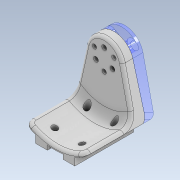
# Autodesk Inventor part: shank_thigh_connector_v3
Saved by Autodesk Inventor 2020 (Build 240168000, 168)
## iProperties
Created: 2021-01-06
Part Number: shank_thigh_connector_v3
Material: PC/ABS Plastic
Document SubType Name: Modeling
Designer: DELL
Density: 0.357273 g/cm^3
Appearance: Clear - Blue
Author: DELL
Autodesk Inventor part; units mm, degrees
ref_plane "YZ Plane" through (0, 0, 0) normal (1, 0, 0) x (0, 1, 0)
ref_plane "XZ Plane" through (0, 0, 0) normal (0, 1, 0) x (-1, 0, 0)
sketch "Sketch1" plane through (0, 0, 0) normal (0, 0, 1) x (1, 0, 0)
  circle A0 centre (0, 0) radius 19
  line L0 (-18.5454, 4.1315) -> (-30, -47.2864)
  line L1 (18.5454, 4.1315) -> (30, -47.2864)
  line L2 (9.9593, -5.75) -> (0, 0) construction
  circle A1 centre (8.4134, -4.8575) radius 2.5
  line L3 (0, 0) -> (9.9593, 5.75) construction
  line L4 (0, 0) -> (-9.9593, -5.75) construction
  circle A2 centre (-8.4134, -4.8575) radius 2.5
  circle A3 centre (0, 0) radius 9.715 construction
  circle A4 centre (0, 0) radius 11.5 construction
  circle A5 centre (0, 9.715) radius 2.5
  line L5 (0, 0) -> (-9.9593, 5.75) construction
  line L6 (11.5, 0) -> (-11.5, 0) construction
  circle A6 centre (-9.9593, 5.75) radius 4
  circle A7 centre (-9.9593, 5.75) radius 2.25
  line L7 (0, -48.5721) -> (0, 22.5) construction
  circle A8 centre (0, -11.5) radius 2.25
  circle A9 centre (0, -11.5) radius 4
  circle A10 centre (9.9593, 5.75) radius 4
  circle A11 centre (9.9593, 5.75) radius 2.25
  arc A12 (-29.0707, -43.1149) -> (29.0707, -43.1149) centre (0, 0) ccw
  arc A13 (-30, -47.2864) -> (30, -47.2864) centre (0, 0) ccw
  line L8 (30, -47.2864) -> (30, -60)
  line L9 (30, -60) -> (-30, -60)
  line L10 (-30, -60) -> (-30, -47.2864)
  line L11 (8, -55.4256) -> (8, -60)
  line L12 (-8, -55.4256) -> (-8, -60)
  line L13 (20, -52.3068) -> (20, -60)
  line L14 (-20, -52.3068) -> (-20, -60)
  point P0 (0, 11.4686)
  point P1 (0, 11.4686)
  point P2 (11.5, 0)
  point P3 (-11.5, 0)
  point P4 (0, -56)
  point P5 (0, -56)
  dimension "d18" = 23
  dimension "d0" = 38
  dimension "d17" = 19.43
  dimension "d19" = 30
  dimension "d20" = 30
  dimension "d21" = 4.5
  dimension "d22" = 8
  dimension "d23" = 5
  dimension "d24" = 104
  dimension "d25" = 112
  dimension "d48" = 60
  dimension "d84" = 16
  dimension "d85" = 4.5744
  dimension "d86" = 22
  dimension "d104" = 60
  dimension "d116" = 40
  constraints: 28 end point, 14 point on circle, 13 centre point, 12 point on line, 10 coincident, 6 equal radius, 6 perpendicular, 2 tangent, 2 vertical, 19 other
  measures "d0" diameter of A0
  measures "d17" diameter of A3
  measures "d19" angle to the sketch x axis of L5
  measures "d20" angle to the sketch x axis of L4
  measures "d21" diameter of A11
  measures "d22" diameter of A10
  measures "d23" diameter of A5
  measures "d24" diameter of A12
  measures "d25" diameter of A13
  measures "d48" distance of L1.end L0.end
  measures "d84" distance between parallel lines of L11 L12
  measures "d85" distance of L11.start L11.end
  measures "d86" distance between parallel lines of L8 L11
  measures "d104" distance from line of A0.centre L9
  measures "d116" distance between parallel lines of L14 L13
extrude "Extrusion1" add sketch "Sketch1" against normal blind 10 contours A0 | A0 L1 A12 L0 | L1 A13 L0 A12 | A1 | A2 | A5 | A6 | A7 | A8 | A9 | A10 | A11
sketch "Sketch4" plane through (0, 0, 0) normal (1, 0, 0) x (0, 1, 0)
  line L0 (4.1315, -10) -> (19, -10) projected
  line L1 (-53, -13) -> (19, -10)
  line L2 (-53, -13) -> (-56, -10)
  line L3 (-53, -13) -> (0, -66)
  line L4 (0, -66) -> (-65, -66)
  line L5 (-65, -66) -> (-65, -1)
  line L6 (4.1315, 0) -> (4.1315, 0) projected
  line L7 (4.1315, 0) -> (4.1315, -10) projected
  line L8 (4.1315, -10) -> (4.1315, -10) projected
  line L9 (4.1315, 0) -> (4.1315, -10) projected
  line L10 (4.1315, 0) -> (-47.2864, 0) projected
  line L11 (-56, -10) -> (-47.2864, -10) projected
  line L12 (-56, -10) -> (19, -10)
  line L13 (-56, 0) -> (-56, -10) projected
  line L14 (-56, -10) -> (-65, -1)
  line L15 (-47.2864, 0) -> (-47.2864, 0) projected
  line L16 (-47.2864, 0) -> (-47.2864, -10) projected
  line L17 (-47.2864, -10) -> (-47.2864, -10) projected
  line L18 (-47.2864, 0) -> (-47.2864, -10) projected
  line L19 (-56, -10) -> (0, -10)
  line L20 (0, -10) -> (0, -66)
  line L21 (19, 0) -> (19, -10) projected
  dimension "d81" = 3
  dimension "d82" = 3
  dimension "d92" = 56
  dimension "d96" = 65
  constraints: 19 end point, 3 collinear, 3 point on line, 2 perpendicular, 1 horizontal
  measures "d81" horizontal distance of L1.start L2.end
  measures "d82" horizontal distance of L1.start L2.end
  measures "d92" distance of L13.end L19.end
  measures "d96" distance between parallel lines of L20 L5
extrude "Extrusion9" add sketch "Sketch4" along normal mid plane 60 contours L0 L1 L20 L12 | L20 L1 L2 L11 L12
extrude "Extrusion10" cut sketch "Sketch1" against normal blind 60 from surface at 0 contours A0 | A0 L1 A12 L0 | L1 A13 L0 A12 | A1 | A2 | A5 | A6 | A7 | A8 | A9 | A10 | A11 keep common part
revolve "Revolution1" cut sketch "Sketch4" angle 360 about axis through (0, 0, -10) along (0, 0, -1) contours L3 L4 L5 L14 L2
sketch "Sketch5" plane through (0, 0, 0) normal (0, 0, 1) x (1, 0, 0)
  arc A0 (-30, -47.2864) -> (30, -47.2864) centre (0, 0) ccw projected
  line L0 (8, -55.4256) -> (8, -60)
  line L1 (-8, -60) -> (-8, -55.4256)
  line L2 (0, 0) -> (0, -56) construction
  line L3 (-8, -60) -> (8, -60)
  line L4 (30, -47.2864) -> (30, -60)
  line L5 (30, -60) -> (8, -60)
  line L6 (-8, -60) -> (-30, -60)
  line L7 (-30, -60) -> (-30, -47.2864)
  line L8 (20, -52.3068) -> (20, -60)
  line L9 (-20, -52.3068) -> (-20, -60)
  line L10 (0, -56) -> (0, -60) construction
  dimension "d93" = 16
  dimension "d94" = 22
  dimension "d95" = 4.5744
  dimension "d105" = 60
  dimension "d117" = 40
  constraints: 22 end point, 5 point on circle, 3 perpendicular, 3 point on line, 3 vertical, 1 horizontal, 1 midpoint, 1 parallel, 2 other
  measures "d93" distance between parallel lines of L0 L1
  measures "d94" distance from line of L4.start L0
  measures "d95" distance of L0.start L0.end
  measures "d105" distance from line of point (0, 0) L3
  measures "d117" distance between parallel lines of L9 L8
extrude "Extrusion14" add sketch "Sketch5" against normal up to surface (10 mm away) contours A0 L1 L6 L9 | A0 L8 L5 L0
extrude "Extrusion11" cut sketch "Sketch1" against normal through all contours A7 | A8 | A11
extrude "Extrusion12" cut sketch "Sketch1" against normal blind 4 contours A1 | A2 | A5
ref_plane "Work Plane1" through (0, 0, -5) normal (0, 0, 1) x (1, 0, 0)
extrude "Extrusion13" cut sketch "Sketch1" against normal blind 15 from surface at -5 contours A6 | A7 | A8 | A9 | A10 | A11
extrude "Extrusion4" add sketch "Sketch1" along normal blind 60 from surface at -10 contours L1 A13 L0 A12 | L13 L9 L11 A13 | A13 L12 L9 L14
fillet "Fillet1" radius 10 1 edges at (0, -52, 0)
fillet "Fillet7" radius 10 2 edges at (-15.2901, -50.8405, -12.91) (15.2901, -50.8405, -12.91)
fillet "Fillet12" radius 6 2 edges at (-29.5354, -45.2006, 50) (29.5354, -45.2006, 50)
fillet "Fillet2" radius 3 5 edges at (-22.6178, -14.1487, 0) (22.6178, -14.1487, 0) (-29.0707, -43.1149, 27) (29.0707, -43.1149, 27) (0, -52, 50)
sketch "Sketch2" plane through (0, 0, 0) normal (0, 1, 0) x (-1, 0, 0)
  line L0 (-2.25, 0) -> (2.25, 0) projected
  line L1 (14, 36.5) -> (-14, 36.5)
  line L2 (-14, 36.5) -> (-14, 3.5)
  line L3 (-14, 3.5) -> (14, 3.5)
  line L4 (14, 3.5) -> (14, 36.5)
  line L5 (14, 36.5) -> (-14, 3.5) construction
  line L6 (-14, 36.5) -> (14, 3.5) construction
  line L7 (8, 50) -> (20, 50) projected
  line L8 (20, -10) -> (20, 50) projected
  line L9 (8, -10) -> (20, -10) projected
  line L10 (8, -10) -> (8, 50) projected
  line L11 (-2.25, -5) -> (2.25, -5) projected
  line L12 (-20, 50) -> (-8, 50) projected
  line L13 (-8, -10) -> (-8, 50) projected
  line L14 (-20, -10) -> (-8, -10) projected
  line L15 (-20, -10) -> (-20, 50) projected
  line L16 (8, 50) -> (20, 50) construction
  line L17 (14, 50) -> (14, -10) construction
  line L18 (-20, -10) -> (-8, -10) construction
  line L19 (-14, -10) -> (-14, 50) construction
  line L20 (-20, 50) -> (-8, 50) construction
  circle A0 centre (14, 3.5) radius 3
  circle A1 centre (14, 3.5) radius 1.75
  circle A2 centre (14, 36.5) radius 3
  circle A3 centre (14, 36.5) radius 1.75
  circle A4 centre (-14, 3.5) radius 3
  circle A5 centre (-14, 3.5) radius 1.75
  circle A6 centre (-14, 36.5) radius 3
  circle A7 centre (-14, 36.5) radius 1.75
  line L21 (0, 54) -> (0, 0) construction
  line L22 (24.3095, 50) -> (-24.3095, 50) projected
  dimension "d120" = 33
  dimension "d121" = 6
  dimension "d122" = 3.5
  dimension "d127" = 28
  dimension "d130" = 13.5
  constraints: 18 end point, 8 centre point, 8 coincident, 6 equal radius, 5 midpoint, 2 parallel, 1 horizontal, 1 perpendicular, 1 point on line, 1 vertical, 2 other
  measures "d120" distance of L1.end L2.end
  measures "d121" diameter of A0
  measures "d122" diameter of A1
  measures "d127" distance of L1.start L1.end
extrude "Extrusion18" cut sketch "Sketch2" against normal through all contours A7 L2 L1 | L1 L2 A7 | A5 L3 L2 | L2 L3 A5 | A3 L4 L1 | L1 L4 A3 | A1 L4 L3 | L3 L4 A1
extrude "Extrusion19" cut sketch "Sketch2" against normal blind 54 contours A6 L2 A7 L1 | L1 A7 L2 A6 | A7 L2 L1 | L1 L2 A7 | A4 L3 A5 L2 | L2 A5 L3 A4 | A2 L4 A3 L1 | L1 A3 L4 A2 | A5 L3 L2 | L2 L3 A5 | A3 L4 L1 | L1 L4 A3 | A0 L4 A1 L3 | L3 A1 L4 A0 | A1 L4 L3 | L3 L4 A1
ref_plane "Work Plane3" through (0, 0, -21) normal (0, 0, 1) x (1, 0, 0)
sketch "Sketch8" plane through (0, 0, -21) normal (0, 0, 1) x (1, 0, 0)
  circle A0 centre (9.9593, 5.75) radius 4 projected
  circle A1 centre (-9.9593, 5.75) radius 4 projected
  circle A2 centre (0, -11.5) radius 4 projected
  line L0 (-18.5454, 4.1315) -> (-28.3857, -40.0401) projected
  arc A3 (18.5454, 4.1315) -> (-18.5454, 4.1315) centre (0, 0) ccw projected
  line L1 (28.3857, -40.0401) -> (18.5454, 4.1315) projected
  line L2 (28.3857, -40.0401) -> (30, -47.2864) projected
  arc A4 (20, -52.3068) -> (30, -47.2864) centre (0, 0) ccw projected
  arc A5 (8, -55.4256) -> (20, -52.3068) centre (0, 0) ccw projected
  arc A6 (-8, -55.4256) -> (8, -55.4256) centre (0, 0) ccw projected
  arc A7 (-20, -52.3068) -> (-8, -55.4256) centre (0, 0) ccw projected
  arc A8 (-30, -47.2864) -> (-20, -52.3068) centre (0, 0) ccw projected
  line L3 (-30, -47.2864) -> (-28.3857, -40.0401) projected
  constraints: 1 horizontal alignment, 4 other
extrude "Extrusion20" add sketch "Sketch8" along normal blind 12 separate body
combine bodies "Combine1" operation type subtract main body 2 bodies to subtract 1 keep tools yes
ref_plane "Work Plane4" through (0, 0, -18) normal (0, 0, -1) x (-1, 0, 0)
sketch "Sketch11" plane through (0, 0, -18) normal (0, 0, -1) x (-1, 0, 0)
  arc A0 (-30, -47.2864) -> (30, -47.2864) centre (0, 0) ccw projected
  line L0 (-5.5, -55.7293) -> (-5.5, 9.2601)
  arc A1 (-5.5, 9.2601) -> (-14.25, 12.5673) centre (-10.5, 9.2601) ccw
  arc A2 (18.5454, 4.1315) -> (-18.5454, 4.1315) centre (0, 0) ccw projected
  line L1 (0, -75.8) -> (0, 34.8) projected
  line L2 (-45.0413, 0) -> (45.0413, 0) projected
  line L3 (5.5, -55.7293) -> (5.5, 9.2601)
  arc A3 (14.25, 12.5673) -> (5.5, 9.2601) centre (10.5, 9.2601) ccw
  point P0 (14.25, 12.5673)
  dimension "d139" = 5
  dimension "d140" = 11
  constraints: 6 point on circle, 4 end point, 4 symmetric about line, 2 centre point, 2 tangent, 1 vertical, 1 other
  measures "d139" radius of A1
  measures "d140" distance between parallel lines of L3 L0
extrude "Extrusion21" cut sketch "Sketch11" against normal through all bodies 2
fillet "Fillet13" radius 4 1 edges at (0, -56, -21)
body "Solid1"
body "Solid2"
